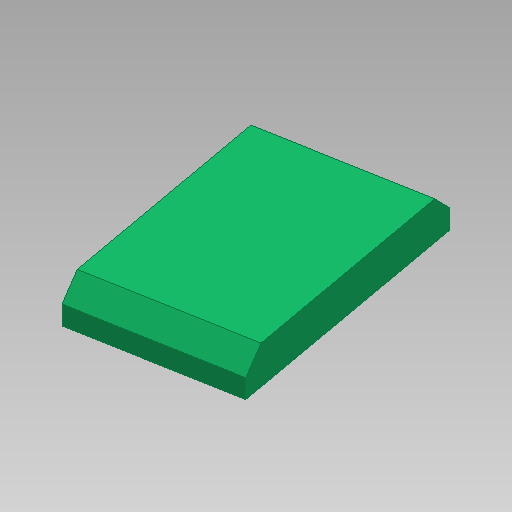
# Autodesk Inventor part: vozik
Saved by Autodesk Inventor 2018.1 (Build 221171000, 171)
## iProperties
Created: 2018-06-23
Part Number: vozik
Material: Všeobecné
Document SubType Name: Modeling
Designer: PS
Density: 1 g/cm^3
Appearance: Výchozí
Author: PS
Autodesk Inventor part; units mm, degrees
ref_plane "YZ Plane" through (0, 0, 0) normal (1, 0, 0) x (0, 1, 0)
ref_plane "XZ Plane" through (0, 0, 0) normal (0, 1, 0) x (-1, 0, 0)
ref_plane "Pracovní rovina1" through (2538.9606, 1040.5981, 0) normal (0, 0, 1) x (-0.177061, 0.9841999, 0)
sketch "Náčrt1" plane through (2538.9606, 1040.5981, 0) normal (0, 0, 1) x (-0.177061, 0.9841999, 0)
  line L0 (3425.3944, 5183.094) -> (-574.6056, 5183.094)
  line L1 (-574.6056, 5183.094) -> (-574.6056, 2683.094)
  line L2 (-574.6056, 2683.094) -> (3425.3944, 2683.094)
  line L3 (3425.3944, 2683.094) -> (3425.3944, 5183.094)
  dimension "d5" = 4000
  dimension "d6" = 2500
  constraints: 8 end point, 2 parallel, 1 coincident, 1 horizontal, 1 perpendicular
  measures "d5" distance of L1.end L2.end
  measures "d6" distance of L0.end L1.end
extrude "Vysunutí1" add sketch "Náčrt1" against normal blind 600
chamfer "Zkosení1" distance 300 angle 45 2 edges at (-1230.2498, -221.3263, 0) (-1938.4939, 3715.4732, 0)
